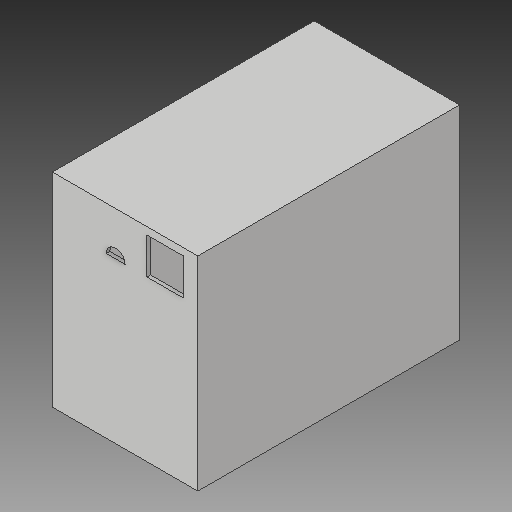
# Autodesk Inventor part: Electronics_Box
Saved by Autodesk Inventor 2018 (Build 220112000, 112)
## iProperties
Created: 2019-07-25
Part Number: Electronics_Box
Material: Generic
Document SubType Name: Modeling
Designer: micha
Density: 1 g/cm^3
Appearance: Default
Author: micha
Autodesk Inventor part; units mm, degrees
ref_plane "YZ Plane" through (0, 0, 0) normal (1, 0, 0) x (0, 1, 0)
ref_plane "XZ Plane" through (0, 0, 0) normal (0, 1, 0) x (-1, 0, 0)
ref_plane "XY Plane" through (0, 0, 0) normal (0, 0, 1) x (1, 0, 0)
sketch "Sketch1" plane through (0, 0, 0) normal (0, 1, 0) x (-1, 0, 0)
  line L0 (0, 0) -> (127, 0)
  line L1 (127, 0) -> (127, -228.6)
  line L2 (127, -228.6) -> (0, -228.6)
  line L3 (0, -228.6) -> (0, 0)
  dimension "d0" = 127
  dimension "d1" = 228.6
  constraints: 8 end point, 2 parallel, 1 horizontal, 1 perpendicular
  measures "d0" distance of L1.end L2.end
  measures "d1" distance of L0.end L1.end
extrude "Extrusion1" add sketch "Sketch1" along normal blind 177.8
sketch "Sketch2" plane through (0, 0, -228.6) normal (0, 0, -1) x (-1, 0, 0)
  line L0 (127, 0) -> (0, 0) projected
  line L1 (127, 0) -> (127, 177.8) projected
  line L2 (0, 177.8) -> (127, 177.8) projected
  line L3 (0, 0) -> (0, 177.8) projected
  line L4 (114.3, 165.1) -> (114.3, 12.7)
  line L5 (114.3, 12.7) -> (12.7, 12.7)
  line L6 (12.7, 12.7) -> (12.7, 165.1)
  line L7 (12.7, 165.1) -> (114.3, 165.1)
  dimension "d4" = 12.7
  constraints: 8 end point, 3 other
  measures "d4" distance between parallel lines of L2 L7
shell "Shell1" thickness 3.175 removed faces 1 at (-84.6667, 59.2667, -228.6)
extrude "Extrusion2" add sketch "Sketch2" against normal blind 3.175
sketch "Sketch3" plane through (-127, 0, 0) normal (0, 0, 1) x (1, 0, 0)
  line L0 (127, 0) -> (127, 177.8) projected
  line L1 (0, 177.8) -> (127, 177.8) projected
  line L2 (114.3, 171.45) -> (82.55, 171.45)
  line L3 (82.55, 171.45) -> (82.55, 139.7)
  line L4 (82.55, 139.7) -> (114.3, 139.7)
  line L5 (114.3, 139.7) -> (114.3, 171.45)
  dimension "d10" = 31.75
  dimension "d11" = 31.75
  dimension "d12" = 6.35
  dimension "d13" = 12.7
  constraints: 8 end point, 2 parallel, 1 horizontal, 1 perpendicular
  measures "d10" distance of L4.end L3.end
  measures "d11" distance of L3.end L2.end
  measures "d12" distance between parallel lines of L2 L1
  measures "d13" distance between parallel lines of L0 L5
extrude "Extrusion3" cut sketch "Sketch3" against normal blind 25.4
sketch "Sketch4" plane through (-127, 0, 0) normal (0, 0, 1) x (1, 0, 0)
  line L0 (46.99, 139.7) -> (63.5, 139.7)
  line L1 (127, 0) -> (127, 177.8) projected
  arc A0 (63.5, 139.7) -> (46.99, 139.7) centre (55.245, 139.7) ccw
  dimension "d16" = 16.51
  dimension "d19" = 63.5
  dimension "d20" = 38.1
  constraints: 2 end point, 2 point on circle, 1 centre point, 1 horizontal, 1 midpoint
  measures "d16" distance of L0.end L0.start
  measures "d19" distance from line of L1 L0.end
  measures "d20" distance from line of L1.end L0
extrude "Extrusion4" cut sketch "Sketch4" against normal blind 25.4
body "Solid1"
